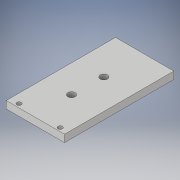
# Autodesk Inventor part: Part100
Saved by Autodesk Inventor 2019.4 (Build 234330000, 330)
## iProperties
Created: 2020-03-03
Part Number: Part100
Material: Generic
Document SubType Name: Modeling
Designer: Niran
Density: 1 g/cm^3
Appearance: Default
Author: Niran
Autodesk Inventor part; units mm, degrees
ref_plane "YZ Plane" through (0, 0, 0) normal (1, 0, 0) x (0, 1, 0)
ref_plane "XZ Plane" through (0, 0, 0) normal (0, 1, 0) x (-1, 0, 0)
ref_plane "XY Plane" through (0, 0, 0) normal (0, 0, 1) x (1, 0, 0)
sketch "Sketch1" plane through (0, 0, 0) normal (0, 1, 0) x (-1, 0, 0)
  line L0 (0, 0) -> (80, 0)
  line L1 (80, 0) -> (80, -150)
  line L2 (80, -150) -> (0, -150)
  line L3 (0, -150) -> (0, 0)
  dimension "d0" = 80
  dimension "d1" = 150
  constraints: 8 end point, 2 parallel, 1 horizontal, 1 perpendicular
  measures "d0" distance of L1.end L2.end
  measures "d1" distance of L0.end L1.end
extrude "Extrusion1" add sketch "Sketch1" along normal blind 10
sketch "Sketch2" plane through (0, 0, 0) normal (0, -1, 0) x (1, 0, 0)
  point P0 (0, 0)
  point P1 (-67.48, -5.0611)
  point P2 (-10.718, -4.8359)
hole "Hole1" at (-67.48, 0, -5.0611) at (-10.718, 0, -4.8359) direction (0, 1, 0) diameter 6 end through all
sketch "Sketch3" plane through (0, 0, 0) normal (0, -1, 0) x (1, 0, 0)
  point P0 (0, 0)
  point P1 (-42.0272, -51.687)
  point P2 (-40.901, -94.9343)
hole "Hole2" at (-42.0272, 0, -51.687) at (-40.901, 0, -94.9343) direction (0, 1, 0) diameter 10 end through all
body "Solid1"
